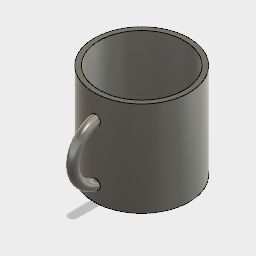
chabei v1 (Autodesk Fusion 360 design; units mm, degrees)
Autodesk Fusion 360 part; units mm, degrees
cylinder "圆柱体基本要素1" add diameter 20 height 20 placed x (1, 0, 0) y (0, 0, -1) z (0, 1, 0) at (0, 0, 0) makes body 1
cylinder "圆柱体基本要素2" add diameter 18 height 20 placed x (1, 0, 0) y (0, 0, -1) z (0, 1, 0) at (20, 0, -30) separate body makes body 2
torus "圆环体基本要素1" add centre line diameter 20 section diameter 2 placed x (1, 0, 0) y (0, 0, -1) z (0, 1, 0) at (20, 0, 50) separate body makes body 3
move_body "MoveFace1" bodies 3 to x (0, -1, 0) y (1, 0, 0) z (0, 0, 1) at (4.4111, 27.3104, 1.4269) on bodies 3
move_body "MoveFace2" bodies 3 to x (1, 0, 0) y (0, 1, 0) z (0, 0, 1) at (-2.398, 3.2082, -23.5297) on bodies 3
delete_face "删除面1" 1 faces at (2.3551, 14.0028, 17.5272) on bodies 3
torus "圆环体基本要素2" add centre line diameter 12 section diameter 2 placed x (1, 0, 0) y (0, 0, -1) z (0, 1, 0) at (-9, 0, -21) separate body makes body 4
move_body "MoveFace3" bodies 4 to x (0, -1, 0) y (1, 0, 0) z (0, 0, 1) at (-29.1073, -14.709, 25.8163) on bodies 4
move_body "MoveFace4" bodies 4 to x (1, 0, 0) y (0, 1, 0) z (0, 0, 1) at (29.313, 14.9926, 3.9667) on bodies 4
combine "合并1" operation add target body 4 tool bodies 1
move_body "对齐1" bodies 4 to x (1, 0, 0) y (0, 1, 0) z (0, 0, 1) at (0, 0, 0)
move_body "对齐2" bodies 4 to x (1, 0, 0) y (0, 1, 0) z (0, 0, 1) at (0, 0, 0)
move_body "对齐3" bodies 2 to x (1, 0, 0) y (0, 1, 0) z (0, 0, 1) at (0, 0, 0)
move_body "对齐4" bodies 4 to x (1, 0, 0) y (0, 1, 0) z (0, 0, 1) at (0, 0, 0)
move_body "对齐5" bodies 4 to x (1, 0, 0) y (0, 1, 0) z (0, 0, 1) at (0, 0, 0)
move_body "对齐6" bodies 2 to x (1, 0, 0) y (0, 1, 0) z (0, 0, 1) at (-20, 0, 30)
move_face "偏移面1" offset -2 1 faces at (-5.1676, 0, -0.3267) on bodies 2
combine "合并2" operation cut target body 4 tool bodies 2
